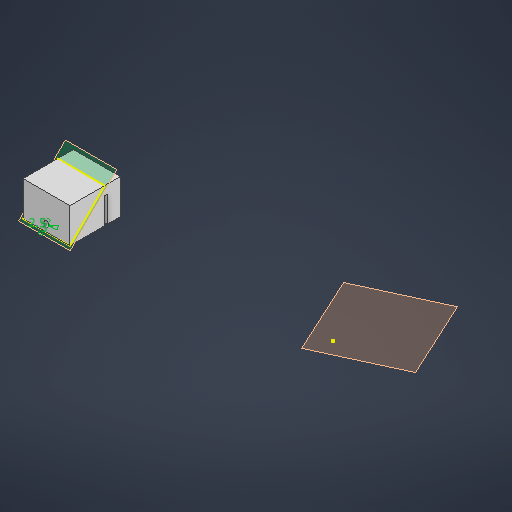
# Autodesk Inventor part: Belt Clip
Saved by Autodesk Inventor 2025.2 (Build 292293000, 293)
## iProperties
Created: 2024-11-19
Part Number: Belt Clip
Material: Generic
Document SubType Name: Modeling
Designer: JL
Density: 1 g/cm^3
Appearance: Default
Author: JL
Autodesk Inventor part; units mm, degrees
ref_plane "YZ Plane" through (0, 0, 0) normal (1, 0, 0) x (0, 1, 0)
ref_plane "Work Plane1" through (-17.0854, 0, -12.1778) normal (0, 1, 0) x (0.4190489, 0, 0.9079637)
sketch "Sketch2" plane through (-17.0854, 0, -12.1778) normal (0, 1, 0) x (0.4190489, 0, 0.9079637)
  line L0 (17.3086, 10.8289) -> (-82.3096, -205.0164) projected
  arc A0 (17.3086, 10.8289) -> (-17.7803, 27.0234) centre (-0.2358, 18.9261) ccw projected
  line L1 (-117.3985, -188.822) -> (-17.7803, 27.0234) projected
  arc A1 (-117.3985, -188.822) -> (-82.3096, -205.0164) centre (-99.8541, -196.9192) ccw projected
  line L2 (-81.4017, -205.4355) -> (18.2166, 10.4099) projected
  arc A2 (-118.3065, -188.4029) -> (-81.4017, -205.4355) centre (-99.8541, -196.9192) ccw projected
  line L3 (-18.6883, 27.4424) -> (-118.3065, -188.4029) projected
  arc A3 (18.2166, 10.4099) -> (-18.6883, 27.4424) centre (-0.2358, 18.9261) ccw projected
  line L4 (-50.7339, -136.6006) -> (-53.0039, -135.553)
  line L5 (-53.0039, -135.553) -> (-51.7467, -132.8291)
  line L6 (-51.7467, -132.8291) -> (-49.4768, -133.8767)
  line L7 (-48.6387, -132.0608) -> (-50.9086, -131.0132)
  line L8 (-50.9086, -131.0132) -> (-49.6515, -128.2893)
  line L9 (-49.6515, -128.2893) -> (-47.3816, -129.3369)
  line L10 (-46.5435, -127.521) -> (-48.8134, -126.4733)
  line L11 (-48.8134, -126.4733) -> (-47.5562, -123.7494)
  line L12 (-47.5562, -123.7494) -> (-45.2863, -124.7971)
  line L13 (-44.4482, -122.9811) -> (-46.7181, -121.9335)
  line L14 (-46.7181, -121.9335) -> (-45.461, -119.2096)
  line L15 (-45.461, -119.2096) -> (-43.1911, -120.2572)
  line L16 (-42.353, -118.4413) -> (-44.6229, -117.3937)
  line L17 (-44.6229, -117.3937) -> (-43.3657, -114.6698)
  line L18 (-43.3657, -114.6698) -> (-41.0958, -115.7174)
  line L19 (-51.572, -138.4165) -> (-58.3818, -135.2737)
  line L20 (-58.3818, -135.2737) -> (-47.0674, -110.7586)
  line L21 (-47.0674, -110.7586) -> (-40.2577, -113.9015)
  line L22 (-53.8419, -137.3689) -> (-53.0039, -135.553) construction
  line L23 (-51.7467, -132.8291) -> (-50.9086, -131.0132) construction
  line L24 (-43.3657, -114.6698) -> (-42.5276, -112.8539) construction
  line L25 (-40.2577, -113.9015) -> (-38.8958, -114.5301) construction
  line L26 (-38.8958, -114.5301) -> (-50.2101, -139.0451)
  line L27 (-50.2101, -139.0451) -> (-32.0508, -147.4261)
  line L28 (-32.0508, -147.4261) -> (-20.7365, -122.9111)
  line L29 (-20.7365, -122.9111) -> (-38.8958, -114.5301)
  point P0 (-48.6387, -132.0608)
  point P1 (-47.3816, -129.3369)
  point P2 (-45.2863, -124.7971)
  point P3 (-44.4482, -122.9811)
  point P4 (-43.1911, -120.2572)
  point P5 (-42.353, -118.4413)
  point P6 (-41.0958, -115.7174)
  dimension "d9" = 2.5
  dimension "d10" = 3
  dimension "d13" = 5
  dimension "d18" = 5
  dimension "d21" = 1.5
  dimension "d22" = 20
  constraints: 52 end point, 9 perpendicular, 8 point on line, 4 collinear, 30 other
  measures "d9" distance of L4.start L4.end
  measures "d10" distance of L4.end L5.end
  measures "d13" distance of L4.start L7.start
  measures "d18" distance between parallel lines of L20 L17
  measures "d21" distance of L21.end L25.end
  measures "d22" distance of L26.end L27.end
ref_plane "Work Plane2" through (-258.0475, 7.5, -40.6457) normal (0, 1, 0) x (0, 0, 1)
ref_plane "Work Plane3" through (-258.0475, 7.5, -40.6457) normal (0, 1, 0) x (0, 0, 1)
extrude "Extrusion2" add sketch "Sketch2" along normal up to surface (7.5 mm away) contours L0 L18 L17 L16 L15 L14 L13 L12 L11 L10 L9 L8 L7 L6 L5 L4 L19 L20 L21 | L29 L28 L27 L26
sketch "Sketch3" plane through (-164.3738, 7.5, -8.5) normal (0, 1, 0) x (1, 0, 0)
  line L0 (27, -29) -> (27, -9) projected
  line L1 (0, 0) -> (27, 0)
  line L2 (27, 0) -> (27, -29)
  line L3 (27, -29) -> (0, -29)
  line L4 (0, -29) -> (0, 0)
  point P0 (164.3738, -8.5)
  constraints: 8 end point, 2 parallel, 1 coincident, 1 horizontal, 1 perpendicular
extrude "Extrusion3" add sketch "Sketch3" along normal blind 5
mirror "Mirror1" about plane through (-150.8738, 0, 10.5) normal (0, -1, 0) of "Extrusion2"
ref_plane "Work Plane4" through (-157.6238, -7.5, 20.5) normal (0, -0.7071068, -0.7071068) x (-1, 0, 0)
sketch "Sketch4" plane through (-157.6238, -7.5, 20.5) normal (0, -0.7071068, -0.7071068) x (-1, 0, 0)
  circle A0 centre (-6.75, 3) radius 1.25
  line L0 (-20.25, 28.2843) -> (6.75, 28.2843) projected
  line L1 (6.75, 28.2843) -> (6.75, 0) projected
  line L2 (6.75, 0) -> (-20.25, 0) projected
  line L3 (-20.25, 0) -> (-20.25, 28.2843) projected
  line L4 (-6.75, 3) -> (-6.75, 0) construction
  point P0 (-157.6238, 19.799)
  dimension "d28" = 2.5
  dimension "d29" = 3
  constraints: 2 end point, 1 centre point, 1 midpoint, 1 perpendicular
  measures "d28" diameter of A0
  measures "d29" distance of L4.start L4.end
extrude "Extrusion4" cut sketch "Sketch4" against normal through all contours A0
extrude "Extrusion5" cut sketch "Sketch4" along normal through all contours A0
body "Solid2"
